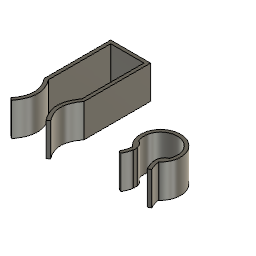
配線抑え (Autodesk Fusion 360 design; units mm, degrees)
Autodesk Fusion 360 part; units mm, degrees
sketch "スケッチ1" plane through (0, 0, 0) normal (0, 0, 1) x (1, 0, 0)
  line L0 (0, 0) -> (12, 0)
  line L1 (12, 0) -> (12, 20)
  line L2 (12, 20) -> (0, 20)
  line L3 (0, 20) -> (0, 0)
  line L4 (1, 19) -> (1, 1)
  line L5 (1, 1) -> (11, 1)
  line L6 (11, 1) -> (11, 19)
  line L7 (11, 19) -> (1, 19)
  spline S0 degree 5 poles (0, 0) (0.1517, -0.2) (0.4418, -0.6) (0.8373, -1.2) (1.2838, -2) (1.6981, -3) (1.9558, -4) (2.044, -5) (1.9558, -6) (1.6981, -7) (1.2838, -8) (0.8373, -8.8) (0.4418, -9.4) (0.1517, -9.8) (0, -10) knots 0 0 0 0 0 0 0.1 0.2 0.3 0.4 0.5 0.6 0.7 0.8 0.9 1 1 1 1 1 1
  spline S1 degree 5 poles (12, 0) (11.8483, -0.2) (11.5582, -0.6) (11.1627, -1.2) (10.7162, -2) (10.3019, -3) (10.0442, -4) (9.956, -5) (10.0442, -6) (10.3019, -7) (10.7162, -8) (11.1627, -8.8) (11.5582, -9.4) (11.8483, -9.8) (12, -10) knots 0 0 0 0 0 0 0.1 0.2 0.3 0.4 0.5 0.6 0.7 0.8 0.9 1 1 1 1 1 1
  spline S2 degree 3 poles (0.7967, 0.6043) (2.0079, -0.9924) (2.8183, -2.6497) (2.9734, -4.4012) (3.1097, -5.9396) (2.6886, -7.4735) (1.902, -8.9122) (1.5893, -9.4841) (1.2196, -10.0468) (0.7967, -10.6043) knots 0 0 0 0 0.448948 0.448948 0.448948 0.843241 0.843241 0.843241 1 1 1 1
  spline S3 degree 3 poles (11.2033, 0.6043) (9.9921, -0.9924) (9.1817, -2.6497) (9.0266, -4.4012) (8.8903, -5.9396) (9.3114, -7.4735) (10.098, -8.9122) (10.4107, -9.4841) (10.7804, -10.0468) (11.2033, -10.6043) knots 0 0 0 0 0.448948 0.448948 0.448948 0.843241 0.843241 0.843241 1 1 1 1
  line L8 (1, 1) -> (1, 0)
  line L9 (11, 1) -> (11, 0)
  line L10 (0, -10) -> (0.7967, -10.6043)
  line L11 (11.2033, -10.6043) -> (12, -10)
  point P0 (2, -5)
  point P1 (10, -5)
  dimension "d1" = 12
  dimension "d2" = 20
  dimension "d3" = -1
  dimension "d4" = -1
  dimension "d5" = 1
  constraint horizontal L0
  constraint vertical L1
  constraint horizontal L2
  constraint vertical L3
  constraint coincident L0.start L3.end
  constraint coincident L0 L8.end
  constraint perpendicular L0 L8
  constraint coincident L0 L9.end
  constraint perpendicular L0 L9
  measures "d1" distance of L0.start L0.end
  measures "d2" distance of L0.start L2.end
extrude "押し出し1" add sketch "スケッチ1" along normal blind 10 contours L0 L1 L2 L3 L4 L6 L7 L8 L9 | L0 S0 S2 L10 | L0 S2 L8 | L0 S3 L9 | L0 S1 S3 L11 makes body 1
sketch "スケッチ2" plane through (0, 0, 0) normal (0, 0, 1) x (1, 0, 0)
  circle A0 centre (35, 0) radius 6
  circle A1 centre (35, 0) radius 5
  spline S0 degree 5 poles (30.4181, -2.0016) (30.5333, -2.064) (30.7542, -2.194) (31.0572, -2.4048) (31.4038, -2.7178) (31.735, -3.1657) (31.9565, -3.6747) (32.0617, -4.2484) (32.0508, -4.8867) (31.932, -5.5849) (31.7152, -6.3378) (31.4705, -6.9797) (31.2495, -7.4819) (31.0859, -7.8258) (31, -8) knots 0 0 0 0 0 0 0.1 0.2 0.3 0.4 0.5 0.6 0.7 0.8 0.9 1 1 1 1 1 1
  spline S1 degree 5 poles (39.5941, -1.9734) (39.4783, -2.0371) (39.2562, -2.1697) (38.9514, -2.3842) (38.6027, -2.7017) (38.269, -3.1544) (38.0453, -3.6673) (37.9385, -4.244) (37.9482, -4.8845) (38.0664, -5.5842) (38.2832, -6.3379) (38.5283, -6.98) (38.7498, -7.4821) (38.9139, -7.8259) (39, -8) knots 0 0 0 0 0 0 0.1 0.2 0.3 0.4 0.5 0.6 0.7 0.8 0.9 1 1 1 1 1 1
  spline S2 degree 3 poles (29.9418, -2.8809) (30.4889, -3.1772) (30.7826, -3.4954) (30.9284, -3.8601) (31.0629, -4.1966) (31.0924, -4.6666) (30.9391, -5.3475) (30.7993, -5.9683) (30.5143, -6.7239) (30.1031, -7.5578) knots 0 0 0 0 0.361862 0.361862 0.361862 0.695661 0.695661 0.695661 1 1 1 1
  spline S3 degree 3 poles (40.0764, -2.8494) (39.5195, -3.156) (39.2187, -3.4846) (39.0709, -3.8598) (38.9348, -4.2054) (38.9075, -4.6846) (39.0657, -5.3737) (39.2071, -5.99) (39.49, -6.7354) (39.8963, -7.5566) knots 0 0 0 0 0.364418 0.364418 0.364418 0.699955 0.699955 0.699955 1 1 1 1
  line L0 (29.9418, -2.8809) -> (29.6547, -2.7253)
  line L1 (40.0764, -2.8494) -> (40.3622, -2.6921)
  line L2 (30.1031, -7.5578) -> (31, -8)
  line L3 (39, -8) -> (39.8963, -7.5566)
  point P0 (32, -4)
  point P1 (38, -4)
  dimension "d8" = 12
  dimension "d9" = -1
  dimension "d10" = 1
  dimension "d11" = -1
  constraint coincident A1 S0.start
  constraint coincident A1 P0
  constraint coincident A1 S1.start
  constraint coincident A1 P1
  constraint coincident A0 L0.end
  constraint coincident A0 L1.end
  measures "d8" diameter of A0
extrude "押し出し2" add sketch "スケッチ2" along normal blind 10 separate body contours A0 A1 S0 S1 S2 S3 L0 L1 | A0 S2 L0 | A0 S3 L1 | A0 S0 S2 L2 | A0 S1 S3 L3 | A1 S0 | A1 S1 makes body 2
